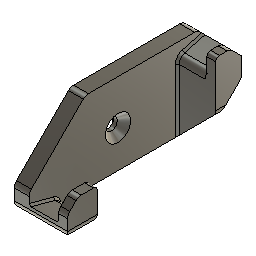
SKADIS_SNS_CalipersHolder (Autodesk Fusion 360 design; units mm, degrees)
Autodesk Fusion 360 part; units mm, degrees
sketch "SlotLayout" plane through (0, 0, 0) normal (1, 0, 0) x (0, 1, 0)
  line L0 (-22.4, 25) -> (-22.4, 15)
  line L1 (82.4, 5) -> (82.4, -5)
  line L2 (-37.6, -5) -> (-37.6, 5)
  line L3 (-80, 5) -> (-80, -5) construction
  line L4 (-97.6, 15) -> (-97.6, 25)
  line L5 (2.4, -5) -> (2.4, 5)
  arc A0 (-77.6, 5) -> (-82.4, 5) centre (-80, 5) ccw
  arc A1 (22.4, 25) -> (17.6, 25) centre (20, 25) ccw
  arc A2 (-97.6, 25) -> (-102.4, 25) centre (-100, 25) ccw
  arc A3 (97.6, 15) -> (102.4, 15) centre (100, 15) ccw
  line L6 (-60, 25) -> (-60, 15) construction
  line L7 (-77.6, -5) -> (-77.6, 5)
  arc A4 (77.6, -5) -> (82.4, -5) centre (80, -5) ccw
  line L8 (-40, 5) -> (-40, -5) construction
  line L9 (-57.6, 15) -> (-57.6, 25)
  line L10 (-62.4, 25) -> (-62.4, 15)
  line L11 (-102.4, 25) -> (-102.4, 15)
  line L12 (97.6, 15) -> (97.6, 25)
  arc A5 (-102.4, 15) -> (-97.6, 15) centre (-100, 15) ccw
  line L13 (20, 25) -> (20, 15) construction
  line L14 (22.4, 25) -> (22.4, 15)
  line L15 (-80, 0) -> (0, 0) construction
  line L16 (62.4, 25) -> (62.4, 15)
  line L17 (42.4, 5) -> (42.4, -5)
  arc A6 (2.5, 5) -> (-2.5, 5) centre (0, 5) ccw
  arc A7 (2.4, 5) -> (-2.4, 5) centre (0, 5) ccw
  line L18 (80, 5) -> (80, -5) construction
  arc A8 (82.4, 5) -> (77.6, 5) centre (80, 5) ccw
  arc A9 (-2.5, -5) -> (2.5, -5) centre (0, -5) ccw
  arc A10 (57.6, 15) -> (62.4, 15) centre (60, 15) ccw
  arc A11 (62.4, 25) -> (57.6, 25) centre (60, 25) ccw
  line L19 (17.6, 15) -> (17.6, 25)
  line L20 (-20, 25) -> (-20, 15) construction
  line L21 (-42.4, 5) -> (-42.4, -5)
  line L22 (60, 25) -> (60, 15) construction
  arc A12 (42.4, 5) -> (37.6, 5) centre (40, 5) ccw
  line L23 (-100, 25) -> (-100, 15) construction
  line L24 (100, 25) -> (100, 15) construction
  arc A13 (-57.6, 25) -> (-62.4, 25) centre (-60, 25) ccw
  arc A14 (37.6, -5) -> (42.4, -5) centre (40, -5) ccw
  line L25 (40, 5) -> (40, -5) construction
  line L26 (-17.6, 15) -> (-17.6, 25)
  arc A15 (-17.6, 25) -> (-22.4, 25) centre (-20, 25) ccw
  line L27 (-82.4, 5) -> (-82.4, -5)
  line L28 (-2.5, 5) -> (-2.5, -5)
  line L29 (-2.4, 5) -> (-2.4, -5)
  line L30 (102.4, 25) -> (102.4, 15)
  arc A16 (17.6, 15) -> (22.4, 15) centre (20, 15) ccw
  arc A17 (-22.4, 15) -> (-17.6, 15) centre (-20, 15) ccw
  line L31 (37.6, -5) -> (37.6, 5)
  line L32 (0, 5) -> (0, -5) construction
  arc A18 (-62.4, 15) -> (-57.6, 15) centre (-60, 15) ccw
  arc A19 (-42.4, -5) -> (-37.6, -5) centre (-40, -5) ccw
  arc A20 (-2.4, -5) -> (2.4, -5) centre (0, -5) ccw
  arc A21 (102.4, 25) -> (97.6, 25) centre (100, 25) ccw
  arc A22 (-82.4, -5) -> (-77.6, -5) centre (-80, -5) ccw
  arc A23 (-37.6, 5) -> (-42.4, 5) centre (-40, 5) ccw
  line L33 (77.6, -5) -> (77.6, 5)
  line L34 (57.6, 15) -> (57.6, 25)
  line L35 (2.5, -5) -> (2.5, 5)
  point P0 (-20, 20)
  point P1 (-40, 0)
  dimension "d9" = -40
  dimension "d10" = 0
  dimension "d255" = 0.1
  dimension "d22" = 10
  dimension "d23" = 2.4
  dimension "d4" = 40
  dimension "d25" = 40
  dimension "d26" = 20
  dimension "d27" = 20
  constraint tangent L27 A22
  constraint tangent L7 A22
  constraint parallel L7 L27
  constraint tangent A0 L7
  constraint tangent A0 L27
  constraint vertical L3
  constraint tangent L21 A19
  constraint tangent L2 A19
  constraint parallel L2 L21
  constraint tangent L2 A23
  constraint tangent L21 A23
  constraint vertical L8
  constraint tangent L29 A20
  constraint tangent L5 A20
  constraint parallel L5 L29
  constraint tangent L5 A7
  constraint tangent A7 L29
  constraint parallel L2 L32
  constraint midpoint L15.start L3
  constraint midpoint L15.end L32
  constraint horizontal L15
  constraint equal L8 L32
  constraint equal L3 L8
  constraint midpoint P1 L8
  constraint coincident P1 L15
  constraint equal A7 A23
  constraint equal A0 A23
  constraint coincident L15.end origin
  constraint symmetric A0.end L1.start L32
  constraint symmetric L1.end L27.end L32
  constraint symmetric L7.start A4.start L32
  constraint symmetric A8.end A0.start L32
  constraint symmetric A4 L32 A22
  constraint symmetric A0 A8 L32
  constraint symmetric L17.start L21.start L32
  constraint symmetric L17.end L21.end L32
  constraint symmetric A14.start L2.start L32
  constraint symmetric A12.end L2.end L32
  constraint symmetric A14 L32 A19
  constraint symmetric A12 L32 A23
  constraint tangent L0 A17
  constraint tangent L26 A17
  constraint parallel L0 L26
  constraint tangent L26 A15
  constraint tangent L0 A15
  constraint vertical L20
  constraint equal L20 L32
  constraint equal A7 A15
  constraint midpoint P0 L20
  constraint symmetric L0.end L14.end L32
  constraint symmetric L26.end A1.end L32
  constraint symmetric L0.start A1.start L32
  constraint symmetric L26.start L19.start L32
  constraint symmetric A1 A15 L32
  constraint symmetric A16 A17 L32
  constraint symmetric A11.end L9.end L32
  constraint symmetric L16.start L10.start L32
  constraint symmetric A11 A13 L32
  constraint symmetric L16.end L10.end L32
  constraint symmetric A10.start L9.start L32
  constraint symmetric A10 L32 A18
  constraint symmetric L12.end L4.end L32
  constraint symmetric L30.start A2.end L32
  constraint symmetric A2 L32 A21
  constraint symmetric A3.end L11.end L32
  constraint symmetric A3.start L4.start L32
  constraint symmetric A3 A5 L32
  measures "d22" distance of A6.centre A9.centre
  measures "d23" radius of A7
  measures "d4" distance of L8 L32
  measures "d25" distance of L3 L8
  measures "d26" horizontal distance of L20.end A6.centre
  measures "d27" vertical distance of P0 L15.end
sketch "VerticalPrintKey" plane through (0, 0, 0) normal (1, 0, 0) x (0, 1, 0)
  line L0 (-2.6, 6.7) -> (2.6, 6.7)
  line L1 (2.6, 6.7) -> (2.6, -6.7)
  line L2 (2.6, -6.7) -> (-2.6, -6.7)
  line L3 (-2.6, -6.7) -> (-2.6, 6.7)
  line L4 (0, 6.7) -> (0, -6.7) construction
  circle A0 centre (0, 0) radius 1.6
  line L5 (2.6, 0) -> (20.8722, 0) construction
  line L6 (20.8722, 0) -> (11.7361, 9.1361) construction
  line L7 (11.7361, 9.1361) -> (11.7361, -9.1361) construction
  line L8 (11.7361, -9.1361) -> (20.8722, 0) construction
  dimension "d18" = 13.4
  dimension "d19" = 5.2
  dimension "d20" = 3.2
  constraint horizontal L0
  constraint vertical L1
  constraint horizontal L2
  constraint vertical L3
  constraint midpoint L0 L4.start
  constraint midpoint L2 L4.end
  constraint midpoint L4 A0.centre
  constraint coincident A0.centre origin
  constraint midpoint L1 L5.start
  constraint perpendicular L1 L5
  constraint perpendicular L5 L7
  constraint perpendicular L6 L8
  constraint midpoint L5 L7
  measures "d18" distance of L4.start L4.end
  measures "d19" distance of L1 L3
  measures "d20" diameter of A0
sketch "HorizontalPrintKey" plane through (0, 0, 0) normal (1, 0, 0) x (0, 1, 0)
  circle A0 centre (0, 0) radius 1.6
  line L0 (2.6, -6.7) -> (-2.6, -6.7)
  line L1 (-2.6, -6.7) -> (-2.6, 6.7)
  line L2 (-2.6, 6.7) -> (2.6, 6.7)
  line L3 (2.6, 6.7) -> (2.6, -6.7)
  line L4 (0, 6.7) -> (0, -6.7) construction
  line L5 (0, 6.7) -> (0, 23.5939) construction
  line L6 (0, 23.5939) -> (-8.4469, 15.1469) construction
  line L7 (-8.4469, 15.1469) -> (8.4469, 15.1469) construction
  line L8 (8.4469, 15.1469) -> (0, 23.5939) construction
  line L9 (17.4, -6.7) -> (17.4, 6.7)
  line L10 (17.4, 6.7) -> (22.6, 6.7)
  line L11 (22.6, -6.7) -> (17.4, -6.7)
  line L12 (22.6, 6.7) -> (22.6, -6.7)
  circle A1 centre (20, 0) radius 1.6
  line L13 (37.4, -6.7) -> (37.4, 6.7)
  line L14 (37.4, 6.7) -> (42.6, 6.7)
  line L15 (42.6, -6.7) -> (37.4, -6.7)
  line L16 (42.6, 6.7) -> (42.6, -6.7)
  circle A2 centre (40, 0) radius 1.6
  line L17 (-37.4, 6.7) -> (-42.6, 6.7)
  line L18 (-22.6, -6.7) -> (-17.4, -6.7)
  line L19 (-42.6, -6.7) -> (-37.4, -6.7)
  line L20 (-37.4, -6.7) -> (-37.4, 6.7)
  circle A3 centre (-40, 0) radius 1.6
  circle A4 centre (-20, 0) radius 1.6
  line L21 (-42.6, 6.7) -> (-42.6, -6.7)
  line L22 (-22.6, 6.7) -> (-22.6, -6.7)
  line L23 (-17.4, -6.7) -> (-17.4, 6.7)
  line L24 (-17.4, 6.7) -> (-22.6, 6.7)
  circle A5 centre (0, 0) radius 3.4
  dimension "d21" = 13.4
  dimension "d24" = 5.2
  dimension "d28" = 3.2
  dimension "d32" = 20
  dimension "d33" = 0
  dimension "d95" = 6.8
  constraint horizontal L2
  constraint vertical L3
  constraint horizontal L0
  constraint vertical L1
  constraint midpoint L4.start L2
  constraint midpoint L4.end L0
  constraint midpoint A0.centre L4
  constraint coincident A0.centre A5.centre
  constraint perpendicular L2 L5
  constraint perpendicular L5 L7
  constraint midpoint L5 L7
  constraint perpendicular L6 L8
  constraint symmetric L5 L9.start L18.end
  constraint symmetric L5 L9.end L23.end
  constraint symmetric L5 L10.end L22.start
  constraint symmetric L5 L11.start L18.start
  constraint symmetric L5 A1 A4
  constraint symmetric L5 L13.start L19.end
  constraint symmetric L5 L13.end L17.start
  constraint symmetric L5 L14.end L17.end
  constraint symmetric L5 L15.start L19.start
  constraint symmetric L5 A2 A3
  measures "d21" distance of L4.end L4.start
  measures "d24" distance of L1 L3
  measures "d28" diameter of A0
  measures "d95" diameter of A5
sketch "MainProfile" plane through (0, 0, 0) normal (1, 0, 0) x (0, 1, 0) in component "SNS_Calipers_150mm"
  line L0 (0, 10) -> (0, -10) construction
  line L1 (17.6, 5.4287) -> (23, 6.8756)
  line L2 (16, 11.6564) -> (16, -10)
  line L3 (17.6, 5.4287) -> (17.6, -10)
  line L4 (23, 5.5) -> (23, 8.5321)
  line L5 (23, 8.5321) -> (16, 6.6564)
  line L6 (23, 5.5) -> (17.6, 0.1)
  line L7 (17.6, -10) -> (0, -10)
  line L8 (17.6, -0.4) -> (16, -0.4)
  line L9 (0, -10) -> (-16, -10)
  line L10 (-16, -8.3436) -> (-24, -6.2)
  line L11 (-24, -7.8564) -> (-16, -10) construction
  line L12 (-24, -7.8564) -> (-24, -3.2)
  line L13 (-16, -10) -> (-21.8564, -10)
  line L14 (-21.8564, -10) -> (-24, -7.8564)
  line L15 (-16, -0.3436) -> (-21.1436, -0.3436)
  line L16 (-10.8, 10) -> (16, 10)
  line L17 (16, 10) -> (21.5321, 10)
  line L18 (21.5321, 10) -> (23, 8.5321)
  line L19 (-24, -3.2) -> (-10.8, 10)
  line L20 (-16, -10) -> (-16, -0.3436)
  line L21 (21.5321, 10) -> (19.8756, 11.6564)
  line L22 (16, 11.6564) -> (19.8756, 11.6564)
  dimension "d36" = 1.6
  dimension "d37" = 1.6
  dimension "d38" = 7
  dimension "d39" = 45
  dimension "d48" = 15
  dimension "d50" = 1.6
  dimension "d51" = 8
  dimension "d52" = 45
  dimension "d53" = 10
  dimension "d54" = 8
  dimension "d55" = 5
  dimension "d56" = 10
  dimension "d58" = 45
  dimension "d59" = 3
  dimension "d60" = 16
  dimension "d62" = 16
  dimension "d63" = 15
  dimension "d64" = 15
  dimension "d74" = 9.6
  dimension "d75" = 0.5
  dimension "d82" = 2.1436
  constraint parallel L2 L3
  constraint coincident L2 L5.end
  constraint vertical L4
  constraint coincident L3 L6.end
  constraint coincident L2.end L7
  constraint horizontal L7
  constraint coincident L0 origin
  constraint coincident L3 L8.start
  constraint coincident L2 L8.end
  constraint perpendicular L2 L8
  constraint perpendicular L0 L9
  constraint coincident L9 L11.end
  constraint coincident L10.start L20
  constraint parallel L10 L11
  constraint coincident L10.end L12
  constraint vertical L12
  constraint vertical L20
  constraint coincident L9.end L11.end
  constraint parallel L9 L13
  constraint perpendicular L12 L15
  constraint coincident L2 L16.end
  constraint perpendicular L2 L16
  constraint coincident L16 L19.end
  constraint coincident L19 L15.end
  constraint vertical L0
  constraint coincident L0.start L16
  constraint perpendicular L0 L16
  constraint perpendicular L18 L19
  constraint collinear L18 L21
  constraint perpendicular L2 L22
  constraint parallel L16 L17
  constraint coincident L4 L5.start
  constraint coincident L4 L1.end
  measures "d36" distance of L1 L5
  measures "d37" distance of L2 L3
  measures "d38" distance of L2 L4.end
  measures "d39" angle of L3 L6
  measures "d48" vertical distance of L5.end L10.start
  measures "d50" distance of L10 L11
  measures "d51" distance of L10.start L15.start
  measures "d52" angle of L13 L14
  measures "d53" distance of L7 origin
  measures "d54" distance of L12 L20
  measures "d55" distance of L5.end L2.start
  measures "d56" distance of L16 origin
  measures "d58" angle of L16 L19
  measures "d59" distance of L10.end L12.end
  measures "d60" distance of L0 L9.end
  measures "d62" distance of L0.end L2.end
  measures "d63" angle of L9 L11
  measures "d64" angle of L1 L7
  measures "d74" distance of L3.end L8
  measures "d75" distance of L6.end L8.start
  measures "d82" vertical distance of L11.start L13.end
extrude "Extrude1" add sketch "MainProfile" along normal blind 4 contours L1 L2 L3 L4 L5 L8 | L1 L3 L4 L6 | L2 L5 L17 L18 | L2 L3 L7 L8 | L2 L7 L9 L15 L16 L19 L20 | L10 L12 L15 L19 L20 | L10 L12 L13 L14 L20 makes body 1 in component "SNS_Calipers_150mm"
extrude "Extrude2" add sketch "MainProfile" along normal blind 8 from surface at 4 contours L1 L2 L3 L4 L5 L8 | L2 L3 L7 L8 | L10 L12 L13 L14 L20 bodies 1 in component "SNS_Calipers_150mm"
extrude "Extrude3" add sketch "MainProfile" along normal blind 2.4 from surface at 12 contours L1 L2 L3 L4 L5 L8 | L1 L3 L4 L6 | L2 L5 L17 L18 | L2 L3 L7 L8 | L2 L17 L21 L22 | L10 L12 L15 L19 L20 | L10 L12 L13 L14 L20 bodies 1 in component "SNS_Calipers_150mm"
chamfer "Chamfer1" distance 10.4 angle 45 1 edges at (14.4, 16.8, -10) on bodies 1 in component "SNS_Calipers_150mm"
chamfer "Chamfer1" distance 2.144 angle 45 1 edges at (14.4, -18.9282, -10) on bodies 1 in component "SNS_Calipers_150mm"
fillet "Fillet2" radius 2 2 edges at (8, 16, 6.6564) (8, -16, -8.3436) on bodies 1 in component "SNS_Calipers_150mm"
fillet "Fillet2" radius 1 2 edges at (13.2, -16, -0.3436) (13.2, 16, 11.6564) on bodies 1 in component "SNS_Calipers_150mm"
fillet "Fillet2" radius 2 8 edges at (13.2, -21.1436, -0.3436) (13.2, -24, -3.2) (13.2, 19.8756, 11.6564) (14.4, 16.95, 0.4) (14.4, -20, -7.856) (14.4, -20, -7.856) (7.1998, -24, -7.8564) (2, 21.5321, 10) on bodies 1 in component "SNS_Calipers_150mm"
fillet "Fillet2" radius 2 4 edges at (2, -24, -3.2) (2, -10.8, 10) (13.2, 23, 5.5) (2, 23, 5.5) on bodies 1 in component "SNS_Calipers_150mm"
chamfer "Chamfer2" distance 0.5 angle 45 10 edges at (4, -20.7412, -7.0732) (4, -16.4133, -8.6607) (4, -16, -9.9391) (12, -20.7412, -7.0732) (12, -16.4133, -8.6607) (4, 20.2412, 7.7929) (4, 16.4133, 6.3393) (4, 16, -2.4391) (12, 20.2412, 7.7929) (12, 16.4133, 6.3393) on bodies 1 in component "SNS_Calipers_150mm"
extrude "Extrude4" cut sketch "HorizontalPrintKey" along normal blind 1.2 contours A0 | L0 L1 L3 A5 | L1 L3 A5 | L1 L2 L3 A5 bodies 1 in component "SNS_Calipers_150mm"
extrude "Extrude5" cut sketch "HorizontalPrintKey" along normal blind 12 contours A0 bodies 1 in component "SNS_Calipers_150mm"
chamfer "Chamfer3" distance 1.8 angle 45 1 edges at (4, -1.4917, 0.5786) on bodies 1 in component "SNS_Calipers_150mm"
sketch "MainProfile (2)" plane through (0, 0, 0) normal (1, 0, 0) x (0, 1, 0) in component "SNS_Calipers_300mm"
  line L0 (0, 12) -> (0, -10) construction
  line L1 (17.6, 7.4287) -> (23, 8.8756)
  line L2 (16, 13.6564) -> (16, -10)
  line L3 (17.6, 7.4287) -> (17.6, -10)
  line L4 (23, 5.5) -> (23, 10.5321)
  line L5 (23, 10.5321) -> (16, 8.6564)
  line L6 (23, 5.5) -> (17.6, 0.1)
  line L7 (17.6, -10) -> (0, -10)
  line L8 (17.6, -0.4) -> (16, -0.4)
  line L9 (0, -10) -> (-16, -10)
  line L10 (-16, -8.3436) -> (-24, -6.2)
  line L11 (-24, -7.8564) -> (-16, -10) construction
  line L12 (-24, -7.8564) -> (-24, -3.2)
  line L13 (-16, -10) -> (-21.8564, -10)
  line L14 (-21.8564, -10) -> (-24, -7.8564)
  line L15 (-16, -0.3436) -> (-21.1436, -0.3436)
  line L16 (-8.8, 12) -> (16, 12)
  line L17 (16, 12) -> (21.5321, 12)
  line L18 (21.5321, 12) -> (23, 10.5321)
  line L19 (-24, -3.2) -> (-8.8, 12)
  line L20 (-16, -10) -> (-16, -0.3436)
  line L21 (21.5321, 12) -> (19.8756, 13.6564)
  line L22 (16, 13.6564) -> (19.8756, 13.6564)
  dimension "d36_1" = 1.6
  dimension "d37_1" = 1.6
  dimension "d38_1" = 7
  dimension "d39_1" = 45
  dimension "d48_1" = 17
  dimension "d50_1" = 1.6
  dimension "d51_1" = 8
  dimension "d52_1" = 45
  dimension "d53_1" = 10
  dimension "d54_1" = 8
  dimension "d55_1" = 5
  dimension "d56_1" = 12
  dimension "d58_1" = 45
  dimension "d59_1" = 3
  dimension "d60_1" = 16
  dimension "d62_1" = 16
  dimension "d63_1" = 15
  dimension "d64_1" = 15
  dimension "d74_1" = 9.6
  dimension "d75_1" = 0.5
  dimension "d82_1" = 2.1436
  constraint parallel L2 L3
  constraint coincident L2 L5.end
  constraint vertical L4
  constraint coincident L3 L6.end
  constraint coincident L2.end L7
  constraint horizontal L7
  constraint coincident L0 origin
  constraint coincident L3 L8.start
  constraint coincident L2 L8.end
  constraint perpendicular L2 L8
  constraint perpendicular L0 L9
  constraint coincident L9 L11.end
  constraint coincident L10.start L20
  constraint parallel L10 L11
  constraint coincident L10.end L12
  constraint vertical L12
  constraint vertical L20
  constraint coincident L9.end L11.end
  constraint parallel L9 L13
  constraint perpendicular L12 L15
  constraint coincident L2 L16.end
  constraint perpendicular L2 L16
  constraint coincident L16 L19.end
  constraint coincident L19 L15.end
  constraint vertical L0
  constraint coincident L0.start L16
  constraint perpendicular L0 L16
  constraint perpendicular L18 L19
  constraint collinear L18 L21
  constraint perpendicular L2 L22
  constraint parallel L16 L17
  constraint coincident L4 L5.start
  constraint coincident L4 L1.end
  measures "d36_1" distance of L1 L5
  measures "d37_1" distance of L2 L3
  measures "d38_1" distance of L2 L4.end
  measures "d39_1" angle of L3 L6
  measures "d48_1" vertical distance of L5.end L10.start
  measures "d50_1" distance of L10 L11
  measures "d51_1" distance of L10.start L15.start
  measures "d52_1" angle of L13 L14
  measures "d53_1" distance of L7 origin
  measures "d54_1" distance of L12 L20
  measures "d55_1" distance of L5.end L2.start
  measures "d56_1" distance of L16 origin
  measures "d58_1" angle of L16 L19
  measures "d59_1" distance of L10.end L12.end
  measures "d60_1" distance of L0 L9.end
  measures "d62_1" distance of L0.end L2.end
  measures "d63_1" angle of L9 L11
  measures "d64_1" angle of L1 L7
  measures "d74_1" distance of L3.end L8
  measures "d75_1" distance of L6.end L8.start
  measures "d82_1" vertical distance of L11.start L13.end
extrude "Extrude1'" add sketch "MainProfile (2)" along normal blind 4 separate body contours L1 L2 L3 L4 L5 L8 | L1 L3 L4 L6 | L2 L5 L17 L18 | L2 L3 L7 L8 | L2 L7 L9 L15 L16 L19 L20 | L10 L12 L15 L19 L20 | L10 L12 L13 L14 L20 makes body 2 in component "SNS_Calipers_300mm"
extrude "Extrude2'" add sketch "MainProfile (2)" along normal blind 8 from surface at 4 contours L1 L2 L3 L4 L5 L8 | L2 L3 L7 L8 | L10 L12 L13 L14 L20 bodies 2 in component "SNS_Calipers_300mm"
extrude "Extrude3'" add sketch "MainProfile (2)" along normal blind 2.4 from surface at 12 contours L1 L2 L3 L4 L5 L8 | L1 L3 L4 L6 | L2 L5 L17 L18 | L2 L3 L7 L8 | L2 L17 L21 L22 | L10 L12 L15 L19 L20 | L10 L12 L13 L14 L20 bodies 2 in component "SNS_Calipers_300mm"
chamfer "Chamfer1'" distance 10.4 angle 45 1 edges at (14.4, 16.8, -10) on bodies 2 in component "SNS_Calipers_300mm"
chamfer "Chamfer1'" distance 2.144 angle 45 1 edges at (14.4, -18.9282, -10) on bodies 2 in component "SNS_Calipers_300mm"
fillet "Fillet2'" radius 2 2 edges at (8, 16, 8.6564) (8, -16, -8.3436) on bodies 2 in component "SNS_Calipers_300mm"
fillet "Fillet2'" radius 1 2 edges at (13.2, -16, -0.3436) (13.2, 16, 13.6564) on bodies 2 in component "SNS_Calipers_300mm"
fillet "Fillet2'" radius 2 8 edges at (13.2, -21.1436, -0.3436) (13.2, -24, -3.2) (13.2, 19.8756, 13.6564) (14.4, 16.95, 0.4) (14.4, -20, -7.856) (14.4, -20, -7.856) (7.1998, -24, -7.8564) (2, 21.5321, 12) on bodies 2 in component "SNS_Calipers_300mm"
fillet "Fillet2'" radius 2 4 edges at (2, -24, -3.2) (2, -8.8, 12) (13.2, 23, 5.5) (2, 23, 5.5) on bodies 2 in component "SNS_Calipers_300mm"
chamfer "Chamfer2'" distance 0.5 angle 45 10 edges at (4, -20.7412, -7.0732) (4, -16.4133, -8.6607) (4, -16, -9.9391) (12, -20.7412, -7.0732) (12, -16.4133, -8.6607) (4, 20.2412, 9.7929) (4, 16.4133, 8.3393) (4, 16, -1.4391) (12, 20.2412, 9.7929) (12, 16.4133, 8.3393) on bodies 2 in component "SNS_Calipers_300mm"
extrude "Extrude4'" cut sketch "HorizontalPrintKey" along normal blind 1.2 contours A0 | L0 L1 L3 A5 | L1 L3 A5 | L1 L2 L3 A5 bodies 2 in component "SNS_Calipers_300mm"
extrude "Extrude5'" cut sketch "HorizontalPrintKey" along normal blind 12 contours A0 bodies 2 in component "SNS_Calipers_300mm"
chamfer "Chamfer3'" distance 1.8 angle 45 1 edges at (4, -1.4917, 0.5786) on bodies 2 in component "SNS_Calipers_300mm"
component "SNS_Calipers_150mm" placed x (1, 0, 0) y (0, 1, 0) z (0, 0, 1) at (0, 0, 0)
component "SNS_Calipers_300mm" placed x (1, 0, 0) y (0, 1, 0) z (0, 0, 1) at (0, 0, 0)
equation "XY_Tolerance = 0.2 mm"
equation "Z_Tolerance = 0.2 mm"
equation "Wall_Thickness = 0.4 mm"
equation "Layer_Height = 0.2 mm"
equation "M3Hole_wClearance = 3.2 mm"
equation "M3Hole_wSelfTapping = 2.8 mm"
equation "d20 = M3Hole_wClearance"
equation "d28 = M3Hole_wClearance"
equation "M3Hole_CounterSink = 1.8 mm"
equation "d50 = d36"
equation "d73 = 8 mm + 2.4 mm"
equation "d74 = 8 mm + 1.6 mm"
equation "d99 = M3Hole_CounterSink"
equation "d50_1 = d36_1"
equation "d73_1 = 8 mm + 2.4 mm"
equation "d74_1 = 8 mm + 1.6 mm"
equation "d99_1 = M3Hole_CounterSink"
named bodies: "CalipersHolder_150mm", "CalipersHolder_300mm"
